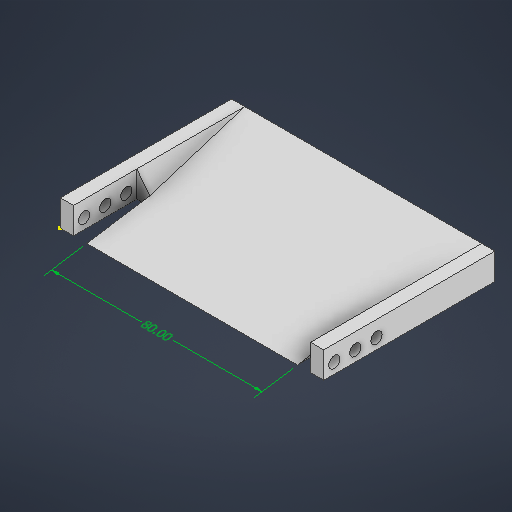
# Autodesk Inventor part: slope
Saved by Autodesk Inventor 2026.1 (Build 301233020, 233B)
## iProperties
Created: 2025-10-28
Part Number: slope
Material: Generic
Document SubType Name: Modeling
Designer: Asus
Density: 1 g/cm^3
Appearance: Default
Author: Asus
Autodesk Inventor part; units mm, degrees
ref_plane "YZ Plane" through (0, 0, 0) normal (1, 0, 0) x (0, 1, 0)
ref_plane "XZ Plane" through (0, 0, 0) normal (0, 1, 0) x (-1, 0, 0)
ref_plane "XY Plane" through (0, 0, 0) normal (0, 0, 1) x (1, 0, 0)
sketch "Sketch1" plane through (0, 0, 0) normal (0, 1, 0) x (-1, 0, 0)
  point P0 (0, 0)
sketch "Sketch2" plane through (0, 0, 0) normal (1, 0, 0) x (0, 1, 0)
  line L0 (0, 0) -> (0, -65)
  line L1 (0, -65) -> (10, -65)
  line L2 (10, -65) -> (0, 0)
  dimension "d0" = 65
  dimension "d2" = 10
  constraints: 6 end point, 1 horizontal, 1 vertical
  measures "d0" distance of L0.start L0.end
  measures "d2" distance of L0.end L1.end
extrude "Extrusion1" add sketch "Sketch2" along normal blind 100
sketch "Sketch3" plane through (100, 0, 0) normal (1, 0, 0) x (0, 0, -1)
  line L0 (65, 10) -> (0, 0) projected
  line L1 (0, 0) -> (24, 0)
  line L2 (24, 0) -> (24, 3.6923)
  line L3 (24, 10) -> (0, 10)
  line L4 (0, 10) -> (0, 0)
  circle A0 centre (4, 4) radius 2.15
  circle A1 centre (12, 4) radius 2.15
  circle A2 centre (20, 4) radius 2.15
  line L5 (24, 10) -> (65, 10)
  line L6 (24, 3.6923) -> (65, 10)
  point P0 (0, 5)
  point P1 (12, 0)
  dimension "d5" = 24
  dimension "d6" = 10
  dimension "d7" = 4.3
  dimension "d9" = 4
  dimension "d10" = 4.3
  dimension "d11" = 8
  dimension "d12" = 4.3
  dimension "d13" = 8
  dimension "d38" = 4
  dimension "d39" = 4
  dimension "d40" = 4
  constraints: 12 end point, 3 centre point, 2 midpoint, 2 parallel, 1 collinear, 1 horizontal, 1 perpendicular, 1 point on line
  measures "d5" distance of L3.end L3.start
  measures "d6" distance of L3.start L1.end
  measures "d7" diameter of A0
  measures "d9" distance from line of L1 A0.centre
  measures "d10" diameter of A1
  measures "d11" distance of A1.centre A0.centre
  measures "d12" diameter of A2
  measures "d13" distance of A1.centre A2.centre
  measures "d38" distance from line of L4 A0.centre
  measures "d39" distance of point (12, 0) A1.centre
  measures "d40" distance from line of L2 A2.centre
sketch "Sketch4" plane through (0, 0, -65) normal (0, -1, 0) x (1, 0, 0)
  line L0 (0, 65) -> (100, 65) projected
  line L1 (85, 65) -> (90, 65)
  line L2 (100, 65) -> (100, 0) projected
  line L3 (85, 65) -> (100, 65)
  line L4 (100, 65) -> (100, 41)
  line L5 (100, 41) -> (90, 41)
  line L6 (100, 41) -> (90, 41)
  line L7 (90, 41) -> (90, 65)
  line L8 (90, 65) -> (100, 65)
  line L9 (100, 65) -> (100, 41)
  dimension "d24" = 10
  constraints: 16 end point, 3 horizontal, 3 parallel, 2 perpendicular, 2 point on line
  measures "d24" distance of L1.end L8.end
extrude "Extrusion2" cut sketch "Sketch4" against normal blind 5
extrude "Extrusion3" add sketch "Sketch3" against normal blind 5 contours L0 A2 A1 L4 L3 L5 | L2 L1 L0 A1 A2
sketch "Sketch5" plane through (0, 0, -65) normal (0, -1, 0) x (1, 0, 0)
  line L0 (0, 65) -> (10, 65)
  line L1 (10, 65) -> (10, 41)
  line L2 (10, 41) -> (0, 41)
  line L3 (0, 41) -> (0, 65)
  dimension "d25" = 10
  dimension "d26" = 24
  constraints: 8 end point, 2 parallel, 1 horizontal, 1 perpendicular
  measures "d25" distance of L1.end L2.end
  measures "d26" distance of L0.end L1.end
extrude "Extrusion4" cut sketch "Sketch5" against normal blind 5
sketch "Sketch6" plane through (0, 0, 0) normal (-1, 0, 0) x (0, 0, 1)
  line L0 (-65, 0) -> (-65, 10) projected
  line L1 (0, 0) -> (-65, 0)
  line L2 (-65, 0) -> (-65, 10)
  line L3 (-65, 10) -> (0, 10)
  line L4 (0, 10) -> (0, 0)
  circle A0 centre (-4, 4) radius 2.15
  circle A1 centre (-12, 4) radius 2.15
  circle A2 centre (-20, 4) radius 2.15
  dimension "d29" = 4.3
  dimension "d30" = 4
  dimension "d31" = 4
  dimension "d32" = 4.3
  dimension "d33" = 8
  dimension "d34" = 4.3
  dimension "d35" = 8
  constraints: 8 end point, 3 centre point, 2 parallel, 1 horizontal, 1 perpendicular
  measures "d29" diameter of A0
  measures "d30" distance from line of L4 A0.centre
  measures "d31" distance from line of L1 A0.centre
  measures "d32" diameter of A1
  measures "d33" distance of A0.centre A1.centre
  measures "d34" diameter of A2
  measures "d35" distance of A1.centre A2.centre
extrude "Extrusion5" add sketch "Sketch6" against normal blind 5
sketch "Sketch7" plane through (10, 0, -24) normal (0, 0, 1) x (1, 0, 0)
  line L0 (-5, 10) -> (85, 10) projected
  line L1 (0, 0) -> (0, 3.6923) projected
  line L2 (-5, 10) -> (0, 3.6923)
  line L3 (-5, 3.6923) -> (0, 3.6923) projected
  line L4 (0, 3.6923) -> (-5, 3.6923)
  line L5 (-5, 3.6923) -> (-5, 10)
  point P0 (-10, 0)
  constraints: 6 end point, 1 collinear, 1 perpendicular
extrude "Extrusion6" add sketch "Sketch7" against normal blind 41
sketch "Sketch8" plane through (90, 0, -24) normal (0, 0, 1) x (1, 0, 0)
  line L0 (0, 3.6923) -> (5, 3.6923) projected
  line L1 (5, 3.6923) -> (5, 10) projected
  line L2 (0, 3.6923) -> (5, 10)
  line L3 (5, 10) -> (5, 3.6923)
  line L4 (5, 3.6923) -> (0, 3.6923)
  point P0 (-90, 0)
  constraints: 6 end point, 1 collinear, 1 perpendicular
extrude "Extrusion7" add sketch "Sketch8" against normal blind 41
body "Solid1"
